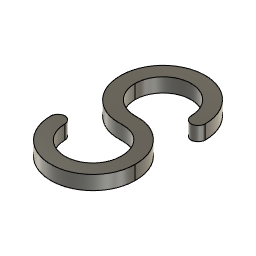
belt hook square v1 (Autodesk Fusion 360 design; units mm, degrees)
Autodesk Fusion 360 part; units mm, degrees
sketch "Sketch1" plane through (0, 0, 0) normal (0, 0, 1) x (1, 0, 0)
  line L0 (20, 30) -> (30, 30) construction
  line L1 (0, 30) -> (20, 30) construction
  arc A0 (20, 30) -> (0, 10) centre (0, 30) ccw
  arc A1 (30, 30) -> (-29.999991, 29.976915) centre (0, 30) ccw
  line L2 (-20, -20) -> (-30, -20) construction
  arc A2 (-20, -20) -> (20, -20) centre (0, -20) ccw
  line L3 (0, -20) -> (-20, -20) construction
  arc A3 (-30, -20) -> (29.999991, -19.977347) centre (0, -20) ccw
  spline S0 degree 5 poles (-30, 30) (-30, 27.543045) (-29.618791, 22.859908) (-27.903261, 16.527353) (-23.619089, 9.544298) (-16.410402, 3.54312) (-8.991104, 0.40546) (-2.530072, -0.269843) (2.725594, 0.310259) (8.561868, -0.689382) (14.460619, -4.261333) (18.158735, -9.330719) (19.665082, -14.254189) (20, -18.00646) (20, -20) knots 0 0 0 0 0 0 0.1 0.2 0.3 0.4 0.5 0.6 0.7 0.8 0.9 1 1 1 1 1 1
  line L4 (20, -10) -> (20, -30)
  line L5 (-30, 40) -> (-30, 20)
  line L6 (-5, 0) -> (5, 0)
  spline S1 degree 5 poles (-20, 30) (-20, 29.999261) (-20, 29.997784) (-19.999999, 29.995569) (-19.999998, 29.992615) (-19.999996, 29.988923) (-19.999994, 29.985969) (-19.999993, 29.983754) (-19.999992, 29.982277) (-19.999991, 29.981539) knots 0 0 0 0 0 0 0.2 0.4 0.6 0.8 1 1 1 1 1 1
  line L7 (-20, 30.001883) -> (-20, 29.998117)
  line L8 (-19.999995, 29.983422) -> (-19.999993, 29.979657)
  spline S2 degree 5 poles (0, 10) (0.550251, 10) (2.23654, 10.004836) (5.153945, 9.964825) (9.748523, 9.274224) (16.410402, 6.45688) (23.61909, 0.455702) (27.903261, -6.527353) (29.618791, -12.859908) (30, -17.543045) (30, -20) knots 0.45104382 0.45104382 0.45104382 0.45104382 0.45104382 0.45104382 0.5 0.6 0.7 0.8 0.9 1 1 1 1 1 1
  line L9 (-3.385738, 10) -> (3.385738, 10)
  line L10 (30, -12.59889) -> (30, -27.40111)
  line L11 (20, 30) -> (30, 30)
  line L12 (-30, -20) -> (-20, -20)
  spline S3 degree 5 poles (20, 30) (20, 29.715656) (20.051763, 29.14684) (20.284676, 28.29323) (20.888717, 27.181271) (22.036643, 25.982954) (23.453028, 25.154234) (25, 24.850713) (26.546972, 25.149338) (27.963358, 25.977131) (29.111284, 27.1775) (29.715324, 28.291885) (29.948237, 29.146594) (30, 29.715656) (30, 30) knots 0 0 0 0 0 0 0.1 0.2 0.3 0.4 0.5 0.6 0.7 0.8 0.9 1 1 1 1 1 1
  line L13 (30, 29) -> (30, 31)
  line L14 (20, 31) -> (20, 29)
  line L15 (23.919554, 25.001605) -> (26.080446, 24.998395)
  spline S4 degree 5 poles (-30, -20) (-30, -19.715656) (-29.94895, -19.146717) (-29.719232, -18.292557) (-29.122246, -17.179385) (-27.980284, -15.980042) (-26.561203, -15.151786) (-25, -14.850713) (-23.438797, -15.151786) (-22.019717, -15.980042) (-20.877754, -17.179385) (-20.280769, -18.292557) (-20.051051, -19.146716) (-20, -19.715656) (-20, -20) knots 0 0 0 0 0 0 0.1 0.2 0.3 0.4 0.5 0.6 0.7 0.8 0.9 1 1 1 1 1 1
  line L16 (-20, -19) -> (-20, -21)
  line L17 (-30, -21) -> (-30, -19)
  arc A4 (-25, -15) -> (-25.013167, -15.000017) centre (-25, -20) ccw
  arc A5 (-30, -20) -> (-30, -20) centre (-25, -20) ccw
  point P0 (0, 10)
  point P1 (25, 25)
  constraint concentric A0 A1
  constraint horizontal L0
  constraint horizontal L1
  constraint coincident L1.start A0.centre
  constraint concentric A2 A3
  constraint coincident A2.centre L3.start
  constraint coincident A0 S1.start
  constraint coincident P0 A0.end
  constraint coincident A3 S2.end
  constraint coincident A1 S0.start
  constraint midpoint A2.end L4
  constraint midpoint S0.start L5
  constraint midpoint origin L6
  constraint midpoint S1.start L7
  constraint midpoint P0 L9
  constraint midpoint S2.end L10
  constraint midpoint L12 A4.centre
  constraint midpoint L0.end L13
  constraint midpoint L0.start L14
  constraint midpoint P1 L15
  constraint midpoint L2.start L16
  constraint tangent A2 L16
  constraint midpoint L2.end L17
  constraint concentric A4 A5
extrude "Extrude1" add sketch "Sketch1" along normal blind 10 contours S1 | A0 A1 A2 A3 S0 S2 L11 L13 L14 L16 L17 A4 A5 | L11 S3 | L12 S4 A4 A5 | L12 A4 A5 picked at (-20, 29.999468) picked at (3.079507, 6.537163) picked at (23.653469, 29.088482) picked at (-23.610921, -19.144586) picked at (-23.388763, -20.739662)
